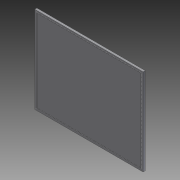
# Autodesk Inventor part: screen
Saved by Autodesk Inventor 2012 (Build 160160000, 160)
## iProperties
Created: 2012-11-23
Part Number: screen
Material: Default
Document SubType Name: Modeling
Designer: r0oland
Density: 1 g/cm^3
Author: r0oland
Autodesk Inventor part; units mm, degrees
ref_plane "YZ Plane" through (0, 0, 0) normal (1, 0, 0) x (0, 1, 0)
ref_plane "XZ Plane" through (0, 0, 0) normal (0, 1, 0) x (-1, 0, 0)
ref_plane "XY Plane" through (0, 0, 0) normal (0, 0, 1) x (1, 0, 0)
sketch "Sketch1" plane through (0, 0, 0) normal (0, 0, 1) x (1, 0, 0)
  line L0 (-250, 200) -> (250, 200)
  line L1 (250, 200) -> (250, -200)
  line L2 (250, -200) -> (-250, -200)
  line L3 (-250, -200) -> (-250, 200)
  line L4 (0, 280) -> (0, -280) projected
  line L5 (-350, 0) -> (350, 0) projected
  point P0 (0, 0)
  dimension "d0" = 500
  dimension "d1" = 400
  constraints: 8 end point, 2 parallel, 1 horizontal, 1 perpendicular, 2 other
  measures "d0" distance of L0.start L0.end
  measures "d1" distance of L2.end L0.start
extrude "Extrusion1" add sketch "Sketch1" along normal blind 10
sketch "Sketch2" plane through (0, 0, 10) normal (0, 0, 1) x (1, 0, 0)
  line L0 (250, 200) -> (250, -200) projected
  line L1 (-250, 200) -> (250, 200) projected
  line L2 (0, 280) -> (0, -280) projected
  line L3 (-350, 0) -> (350, 0) projected
  line L4 (-240, 190) -> (240, 190)
  line L5 (240, 190) -> (240, -190)
  line L6 (240, -190) -> (-240, -190)
  line L7 (-240, -190) -> (-240, 190)
  point P0 (0, 0)
  point P1 (-240, 0)
  point P2 (0, 190)
  dimension "d4" = 10
  dimension "d5" = 10
  constraints: 8 end point, 2 midpoint, 2 parallel, 1 horizontal, 1 horizontal alignment, 1 perpendicular, 1 vertical alignment
  measures "d4" distance between parallel lines of L1 L4
  measures "d5" distance between parallel lines of L0 L5
extrude "Extrusion2" cut sketch "Sketch2" against normal blind 2 contours L5 L6 L2 L3 | L3 L2 L4 L5 | L2 L3 L7 L4 | L2 L6 L7 L3
body "Solid1"
